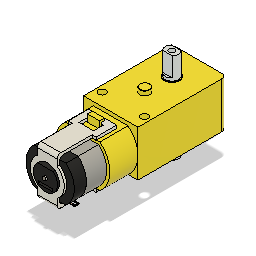
BO DC Motor (Autodesk Fusion 360 design; units mm, degrees)
Autodesk Fusion 360 part; units mm, degrees
sketch "Cylinder profile" plane through (0, 0, 0) normal (0, 1, 0) x (1, 0, 0) in component "Motor Shaft"
  circle A0 centre (0, 0) radius 2.73
  dimension "d6" = 5.46
  measures "d6" diameter of A0
extrude "Extrude1" add sketch "Cylinder profile" along normal mid plane 37.42 makes body 1 in component "Motor Shaft"
sketch "Shaft Cut profile" plane through (0, 18.71, 0) normal (0, 1, 0) x (-1, 0, 0) in component "Motor Shaft"
  circle A0 centre (0, 0) radius 2.73
  line L0 (2.0076, -1.85) -> (-2.0076, -1.85)
  line L1 (0, 0) -> (2.73, 0) construction
  line L2 (2.0076, 1.85) -> (-2.0076, 1.85)
  circle A1 centre (0, 0) radius 1.18
  point P0 (2.73, 0)
  dimension "d9" = 1.85
  dimension "d15" = 2.36
  measures "d9" distance of A0.centre L0
  measures "d15" diameter of A1
extrude "Extrude2" cut sketch "Shaft Cut profile" against normal blind 7.96 contours A0 L2 | A0 L0 bodies 1 in component "Motor Shaft"
extrude "Extrude3" cut sketch "Shaft Cut profile" along normal blind 7.96 from surface at -37.42 contours A0 L2 | A0 L0 bodies 1 in component "Motor Shaft"
extrude "Extrude4" cut sketch "Shaft Cut profile" against normal blind 5.96 contours A1 bodies 1 in component "Motor Shaft"
extrude "Extrude5" cut sketch "Shaft Cut profile" along normal blind 5.96 from surface at -37.42 contours A1 bodies 1 in component "Motor Shaft"
sketch "Case only cross section" plane through (0, 0, 0) normal (0, 1, 0) x (1, 0, 0) in component "Motor Casing"
  circle A0 centre (0, 0) radius 2.73
  line L0 (2.0076, 1.85) -> (-2.0076, 1.85) construction
  line L1 (-2.0076, -1.85) -> (2.0076, -1.85) construction
  line L2 (11.25, 11.33) -> (-11.25, 11.33)
  line L3 (-11.25, 11.33) -> (-11.25, -25.27)
  line L4 (-11.25, -25.27) -> (11.25, -25.27)
  line L5 (11.25, -25.27) -> (11.25, 11.33)
  line L6 (11.25, 11.33) -> (-11.25, -25.27) construction
  line L7 (-11.25, 11.33) -> (11.25, -25.27) construction
  line L8 (0, 9) -> (0, -17) construction
  line L9 (10.25, -21.61) -> (7.25, -21.61) construction
  line L10 (7.25, -21.61) -> (7.25, -18.61) construction
  line L11 (7.25, -18.61) -> (10.25, -18.61) construction
  line L12 (10.25, -18.61) -> (10.25, -21.61) construction
  line L13 (10.25, -21.61) -> (7.25, -18.61) construction
  line L14 (7.25, -21.61) -> (10.25, -18.61) construction
  circle A1 centre (8.75, -20.11) radius 1.5
  circle A2 centre (-8.75, -20.11) radius 1.5
  point P0 (0, -6.97)
  point P1 (8.75, -20.11)
  dimension "d22" = 5.46
  dimension "d37" = 36.6
  dimension "d38" = 22.5
  dimension "d39" = 9.48
  dimension "d41" = 3
  dimension "d42" = 3
  dimension "d44" = 6.66
  dimension "d45" = 4
  dimension "d46" = 3
  measures "d22" diameter of A0
  measures "d37" distance of L2.end L3.end
  measures "d38" distance of L3.end L4.end
  measures "d39" distance of L0 L2
  measures "d41" distance of L10.end L11.end
  measures "d42" distance of L9.end L10.end
  measures "d44" distance of L4 L11
  measures "d45" distance of L5 L10
  measures "d46" diameter of A1
extrude "Extrude1'" add sketch "Case only cross section" along normal mid plane 18.94 separate body makes body 2 in component "Motor Casing"
sketch "Protrusion (wheel side)" plane through (0, 9.47, 0) normal (0, 1, 0) x (-1, 0, 0) in component "Motor Casing"
  circle A0 centre (0, 0) radius 2.73
  circle A1 centre (-8.75, 20.11) radius 1.5
  circle A2 centre (8.75, 20.11) radius 1.5
  line L0 (-11.25, 25.27) -> (-11.25, -11.33)
  line L1 (-11.25, -11.33) -> (11.25, -11.33)
  line L2 (11.25, -11.33) -> (11.25, 25.27)
  line L3 (11.25, 25.27) -> (-11.25, 25.27)
  line L4 (0, -5) -> (0, 13) construction
  line L5 (-2.08, 9.14) -> (2.08, 9.14) construction
  line L6 (2.08, 9.14) -> (2.08, 13.3) construction
  line L7 (2.08, 13.3) -> (-2.08, 13.3) construction
  line L8 (-2.08, 13.3) -> (-2.08, 9.14) construction
  line L9 (-2.08, 9.14) -> (2.08, 13.3) construction
  line L10 (2.08, 9.14) -> (-2.08, 13.3) construction
  line L11 (2.0076, 1.85) -> (-2.0076, 1.85) construction
  circle A3 centre (0, 11.22) radius 2.08
  point P0 (0, 11.22)
  dimension "d50" = 4.16
  dimension "d51" = 4.16
  dimension "d52" = 11.45
  dimension "d53" = 4.16
  measures "d50" distance of L6.end L7.end
  measures "d51" distance of L5.end L6.end
  measures "d52" distance of L7 L11
  measures "d53" diameter of A3
extrude "Extrude2'" add sketch "Protrusion (wheel side)" along normal blind 1.9 contours A3 bodies 2 in component "Motor Casing"
sketch "Casing notch" plane through (0, 0, 0) normal (0, 1, 0) x (1, 0, 0) in component "Motor Casing"
  line L0 (-2.5, 16.53) -> (2.5, 16.53)
  line L1 (2.5, 16.53) -> (2.5, 11.33)
  line L2 (2.5, 11.33) -> (-2.5, 11.33)
  line L3 (-2.5, 11.33) -> (-2.5, 16.53)
  line L4 (11.25, 11.33) -> (-11.25, 11.33) construction
  line L5 (1.5, 12.43) -> (-1.5, 12.43) construction
  line L6 (-1.5, 12.43) -> (-1.5, 15.43) construction
  line L7 (-1.5, 15.43) -> (1.5, 15.43) construction
  line L8 (1.5, 15.43) -> (1.5, 12.43) construction
  line L9 (1.5, 12.43) -> (-1.5, 15.43) construction
  line L10 (-1.5, 12.43) -> (1.5, 15.43) construction
  circle A0 centre (0, 13.93) radius 1.5
  point P0 (0, 13.93)
  dimension "d56" = 5
  dimension "d57" = 5.2
  dimension "d58" = 2.5
  dimension "d60" = 3
  dimension "d61" = 3
  dimension "d62" = 1.1
  dimension "d64" = 3
  measures "d56" distance of L0.start L0.end
  measures "d57" distance of L0.start L2.end
  measures "d58" distance of origin L1
  measures "d60" distance of L6.end L7.end
  measures "d61" distance of L5.end L6.end
  measures "d62" distance of L0 L7
  measures "d64" diameter of A0
extrude "Extrude3'" add sketch "Casing notch" along normal mid plane 3 bodies 2 in component "Motor Casing"
sketch "Motor casing" plane through (0, 0, 25.27) normal (0, 0, 1) x (1, 0, 0) in component "Motor Casing"
  line L0 (11.25, -9.47) -> (11.25, 9.47)
  line L1 (11.25, 9.47) -> (-11.25, 9.47)
  line L2 (-11.25, 9.47) -> (-11.25, -9.47)
  line L3 (-11.25, -9.47) -> (11.25, -9.47)
  line L4 (7.1325, -9.47) -> (-7.1325, -9.47)
  line L5 (0, -0.77) -> (-8, -0.77) construction
  line L6 (7.1325, 7.93) -> (-7.1325, 7.93)
  arc A0 (7.1325, -9.47) -> (7.1325, 7.93) centre (0, -0.77) ccw
  arc A1 (-7.1325, 7.93) -> (-7.1325, -9.47) centre (0, -0.77) ccw
  line L7 (-6.5385, 6.73) -> (6.5385, 6.73)
  line L8 (-6.5385, -8.27) -> (6.5385, -8.27)
  arc A2 (6.5385, -8.27) -> (6.5385, 6.73) centre (0, -0.77) ccw
  arc A3 (-6.5385, 6.73) -> (-6.5385, -8.27) centre (0, -0.77) ccw
  dimension "d74" = 8.7
  dimension "d75" = 11.25
  dimension "d76" = 11.25
  dimension "d82" = 15
  dimension "d83" = 7.5
  dimension "d84" = 9.95
  measures "d74" distance of L5.start L4
  measures "d75" radius of A0
  measures "d76" radius of A1
  measures "d82" distance of L7 L8
  measures "d83" distance of L5.start L8
  measures "d84" radius of A2
extrude "Extrude4'" add sketch "Motor casing" along normal blind 11.6 contours L3 L4 L6 A0 A1 bodies 2 in component "Motor Casing"
sketch "Motor casing rect cutout" plane through (0, 7.93, 0) normal (0, 1, 0) x (-1, 0, 0) in component "Motor Casing"
  line L0 (-7.1325, 25.27) -> (7.1325, 25.27)
  line L1 (7.1325, 25.27) -> (7.1325, 36.87)
  line L2 (7.1325, 36.87) -> (-7.1325, 36.87)
  line L3 (-7.1325, 36.87) -> (-7.1325, 25.27)
  line L4 (-3, 28.87) -> (3, 28.87)
  line L5 (3, 28.87) -> (3, 31.37)
  line L6 (3, 31.37) -> (-3, 31.37)
  line L7 (-3, 31.37) -> (-3, 28.87)
  line L8 (-3, 28.87) -> (3, 31.37) construction
  line L9 (3, 28.87) -> (-3, 31.37) construction
  point P0 (0, 30.12)
  dimension "d90" = 6
  dimension "d91" = 2.5
  dimension "d92" = 3.6
  measures "d90" distance of L5.end L6.end
  measures "d91" distance of L4.end L5.end
  measures "d92" distance of L0 L4
extrude "Extrude5'" cut sketch "Motor casing rect cutout" against normal blind 17.4 contours L4 L5 L6 L7 bodies 2 in component "Motor Casing"
sketch "Motor casing Latch" plane through (0, 0, 0) normal (1, 0, 0) x (0, 0, -1) in component "Motor Casing"
  line L0 (-28.87, 7.93) -> (-31.37, 7.93) construction
  line L1 (-31.37, 7.93) -> (-32.37, 7.93)
  line L2 (-31.37, 7.93) -> (-31.37, 9.93)
  line L3 (-31.37, 9.93) -> (-30.37, 9.93)
  line L4 (-30.37, 9.93) -> (-30.37, 10.93)
  line L5 (-30.37, 10.93) -> (-32.37, 10.93)
  line L6 (-32.37, 10.93) -> (-32.37, 7.93)
  line L7 (-31.37, -9.47) -> (-28.87, -9.47) construction
  line L8 (-31.37, -9.47) -> (-32.37, -9.47)
  line L9 (-31.37, -9.47) -> (-31.37, -11.47)
  line L10 (-31.37, -11.47) -> (-30.37, -11.47)
  line L11 (-30.37, -11.47) -> (-30.37, -12.47)
  line L12 (-30.37, -12.47) -> (-32.37, -12.47)
  line L13 (-32.37, -12.47) -> (-32.37, -9.47)
  dimension "d103" = 1
  dimension "d104" = 2
  dimension "d105" = 1
  dimension "d106" = 1
  dimension "d107" = 2
  dimension "d108" = 1
  dimension "d109" = 2
  dimension "d110" = 1
  dimension "d111" = 1
  dimension "d112" = 2
  measures "d103" distance of L0.end L1.end
  measures "d104" distance of L0.end L2.end
  measures "d105" distance of L2.end L3.end
  measures "d106" distance of L3.end L4.end
  measures "d107" distance of L4.end L5.end
  measures "d108" distance of L7.start L8.end
  measures "d109" distance of L7.start L9.end
  measures "d110" distance of L9.end L10.end
  measures "d111" distance of L10.end L11.end
  measures "d112" distance of L11.end L12.end
extrude "Extrude6" add sketch "Motor casing Latch" along normal mid plane 5 bodies 2 in component "Motor Casing"
fillet "Fillet1" radius 2 2 edges at (-11.25, 0, -11.33) (11.25, 0, -11.33) on bodies 2 in component "Motor Casing"
fillet "Fillet2" radius 1 2 edges at (2.5, 0, -11.33) (-2.5, 0, -11.33) on bodies 2 in component "Motor Casing"
sketch "Motor cross section" plane through (0, 0, 25.27) normal (0, 0, 1) x (1, 0, 0) in component "Driving Motor"
  line L0 (-6.5385, -8.27) -> (6.5385, -8.27)
  arc A0 (6.5385, -8.27) -> (6.5385, 6.73) centre (0, -0.77) ccw
  line L1 (6.5385, 6.73) -> (-6.5385, 6.73)
  arc A1 (-6.5385, 6.73) -> (-6.5385, -8.27) centre (0, -0.77) ccw
extrude "Extrude1''" add sketch "Motor cross section" along normal blind 25 separate body makes body 3 in component "Driving Motor"
ref_plane "WorkPlane1" through (0, -0.77, 45.27) normal (0, 0, 1) x (1, 0, 0) in component "Driving Motor"
split "Split1" by plane through (0, -0.77, 45.27) normal (0, 0, 1) bodies 3 makes body 4 at (1.8819, 0.3568, 50.27) in component "Driving Motor"
sketch "ECT section" plane through (0, -8.27, 0) normal (0, -1, 0) x (1, 0, 0) in component "Driving Motor"
  line L0 (-6.5385, 45.27) -> (6.5385, 45.27) construction
  line L1 (6.5385, 45.27) -> (6.5385, 50.27) construction
  line L2 (6.5385, 50.27) -> (-6.5385, 50.27) construction
  line L3 (-6.5385, 50.27) -> (-6.5385, 45.27) construction
  line L4 (-6.5385, 50.27) -> (6.5385, 45.27) construction
  line L5 (-6.5385, 45.27) -> (6.5385, 50.27) construction
  line L6 (8.6, 48.77) -> (-8.6, 48.77)
  line L7 (-8.6, 48.77) -> (-8.6, 46.77)
  line L8 (-8.6, 46.77) -> (8.6, 46.77)
  line L9 (8.6, 46.77) -> (8.6, 48.77)
  line L10 (8.6, 48.77) -> (-8.6, 46.77) construction
  line L11 (-8.6, 48.77) -> (8.6, 46.77) construction
  line L12 (8.1, 48.27) -> (6.1, 48.27)
  line L13 (6.1, 48.27) -> (6.1, 47.27)
  line L14 (6.1, 47.27) -> (8.1, 47.27)
  line L15 (8.1, 47.27) -> (8.1, 48.27)
  line L16 (8.1, 48.27) -> (6.1, 47.27) construction
  line L17 (6.1, 48.27) -> (8.1, 47.27) construction
  line L18 (0, 45.9618) -> (0, 49.5782) construction
  line L19 (-6.1, 47.27) -> (-8.1, 47.27)
  line L20 (-8.1, 47.27) -> (-8.1, 48.27)
  line L21 (-8.1, 48.27) -> (-6.1, 48.27)
  line L22 (-6.1, 48.27) -> (-6.1, 47.27)
  point P0 (0, 47.77)
  point P1 (7.1, 47.77)
  dimension "d129" = 17.2
  dimension "d130" = 2
  dimension "d132" = 1
  dimension "d133" = 2
  dimension "d134" = 0.5
  measures "d129" distance of L7.end L8.end
  measures "d130" distance of L6.end L7.end
  measures "d132" distance of L12.end L13.end
  measures "d133" distance of L13.end L14.end
  measures "d134" distance of L9 L15
extrude "Extrude2''" add sketch "ECT section" along normal blind 0.25 separate body makes body 5 in component "Driving Motor"
sketch "Motor bottom extension" plane through (0, 0, 50.27) normal (0, 0, 1) x (1, 0, 0) in component "Driving Motor"
  arc A0 (-6.5385, 6.73) -> (-6.5385, -8.27) centre (0, -0.77) ccw construction
  line L0 (-6.5385, -8.27) -> (6.5385, -8.27) construction
  arc A1 (6.5385, -8.27) -> (6.5385, 6.73) centre (0, -0.77) ccw construction
  line L1 (6.5385, 6.73) -> (-6.5385, 6.73) construction
  line L2 (3.2261, 3.05) -> (-3.2261, 3.05)
  arc A2 (-3.2261, 3.05) -> (3.2261, 3.05) centre (0, -0.77) ccw
  line L3 (3, -3.22) -> (-3, -3.22)
  line L4 (-3, -3.22) -> (-3, -4.22)
  line L5 (-3, -4.22) -> (3, -4.22)
  line L6 (3, -4.22) -> (3, -3.22)
  line L7 (3, -3.22) -> (-3, -4.22) construction
  line L8 (-3, -3.22) -> (3, -4.22) construction
  circle A3 centre (0, -0.77) radius 0.75
  point P0 (0, -3.72)
  dimension "d141" = 10
  dimension "d142" = 3.82
  dimension "d143" = 6
  dimension "d144" = 1
  dimension "d145" = 3.45
  dimension "d146" = 1.5
  measures "d141" diameter of A2
  measures "d142" distance of A0.centre L2
  measures "d143" distance of L4.end L5.end
  measures "d144" distance of L3.end L4.end
  measures "d145" distance of A0.centre L5
  measures "d146" diameter of A3
extrude "Extrude3''" add sketch "Motor bottom extension" along normal blind 2 bodies 4 in component "Driving Motor"
extrude "Extrude4''" add 1 faces at (0.3665, -0.77, 50.27) along direction (0, 0, 1) blind 2.5 separate body on bodies 4 makes body 6 in component "Driving Motor"
sketch "Motor Belt (Top)" plane through (0, 7.93, 0) normal (0, 1, 0) x (-1, 0, 0) in component "Fasteners"
  line L0 (-2.5, 31.37) -> (-2.5, 32.37)
  line L1 (-2.5, 32.37) -> (2.5, 32.37) construction
  line L2 (2.5, 32.37) -> (2.5, 31.37)
  line L3 (2.5, 31.37) -> (3, 31.37) construction
  line L4 (3, 31.37) -> (3, 28.87) construction
  line L5 (3, 28.87) -> (-3, 28.87) construction
  line L6 (-3, 28.87) -> (-3, 31.37) construction
  line L7 (-3, 31.37) -> (-2.5, 31.37) construction
  line L8 (-5.75, 28.57) -> (5.75, 28.57)
  line L9 (5.75, 28.57) -> (5.75, 37.07)
  line L10 (-5.75, 37.07) -> (-5.75, 28.57)
  line L11 (-5.75, 28.57) -> (5.75, 37.07) construction
  line L12 (5.75, 28.57) -> (-5.75, 37.07) construction
  line L13 (3, 31.37) -> (-3, 31.37) construction
  line L14 (3, 31.37) -> (-3, 31.37)
  line L15 (-3, 31.37) -> (-3, 35.37)
  line L16 (-3, 35.37) -> (3, 35.37)
  line L17 (3, 35.37) -> (3, 31.37)
  line L18 (-3, 28.87) -> (-3, 31.37) construction
  line L19 (3, 28.87) -> (-3, 28.87) construction
  line L20 (3, 31.37) -> (3, 28.87) construction
  line L21 (4.1, 37.07) -> (4.1, 51.47)
  line L22 (4.1, 51.47) -> (-4.1, 51.47)
  line L23 (-4.1, 51.47) -> (-4.1, 37.07)
  line L24 (-4.1, 37.07) -> (4.1, 51.47) construction
  line L25 (4.1, 37.07) -> (-4.1, 51.47) construction
  line L26 (5.75, 37.07) -> (4.1, 37.07)
  line L27 (-4.1, 37.07) -> (-5.75, 37.07)
  point P0 (0, 32.82)
  point P1 (0, 44.27)
  dimension "d154" = 11.5
  dimension "d155" = 8.5
  dimension "d156" = 0.3
  dimension "d157" = 6
  dimension "d158" = 4
  dimension "d159" = 8.2
  dimension "d160" = 14.4
  measures "d154" distance of L9.end L10.start
  measures "d155" distance of L8.end L9.end
  measures "d156" distance of L5 L8
  measures "d157" distance of L3.end L6.end
  measures "d158" distance of L3.end L16.end
  measures "d159" distance of L21.end L22.end
  measures "d160" distance of L21.start L21.end
sketch "Motor Belt (Bottom)" plane through (0, -9.47, 0) normal (0, -1, 0) x (1, 0, 0) in component "Fasteners"
  line L0 (2.5, 32.37) -> (2.5, 31.37) construction
  line L1 (2.5, 31.37) -> (3, 31.37) construction
  line L2 (3, 31.37) -> (3, 28.87) construction
  line L3 (3, 28.87) -> (-3, 28.87) construction
  line L4 (-3, 28.87) -> (-3, 31.37) construction
  line L5 (-3, 31.37) -> (-2.5, 31.37) construction
  line L6 (-2.5, 31.37) -> (-2.5, 32.37) construction
  line L7 (-2.5, 32.37) -> (2.5, 32.37) construction
  line L8 (5.75, 37.07) -> (5.75, 28.57)
  line L9 (4.1, 51.47) -> (4.1, 37.07)
  line L10 (-4.1, 51.47) -> (4.1, 51.47)
  line L11 (-4.1, 37.07) -> (-4.1, 51.47)
  line L12 (-5.75, 37.07) -> (-4.1, 37.07)
  line L13 (-5.75, 28.57) -> (-5.75, 37.07)
  line L14 (5.75, 28.57) -> (-5.75, 28.57)
  line L15 (4.1, 37.07) -> (5.75, 37.07)
  line L16 (3, 35.37) -> (-3, 35.37)
  line L17 (-3, 35.37) -> (-3, 31.37)
  line L18 (3, 31.37) -> (3, 35.37)
  line L19 (-3, 31.37) -> (3, 31.37)
sketch "ECT Spacer base" plane through (0, -8.52, 0) normal (0, -1, 0) x (1, 0, 0) in component "Fasteners"
  line L0 (4.07, 48.77) -> (-4.07, 48.77)
  line L1 (-4.07, 48.77) -> (-4.07, 45.77)
  line L2 (-4.07, 45.77) -> (4.07, 45.77)
  line L3 (4.07, 45.77) -> (4.07, 48.77)
  line L4 (4.07, 48.77) -> (-4.07, 45.77) construction
  line L5 (-4.07, 48.77) -> (4.07, 45.77) construction
  line L6 (8.6, 48.77) -> (-8.6, 48.77) construction
  point P0 (0, 47.27)
  dimension "d161" = 8.14
  dimension "d162" = 3
  measures "d161" distance of L1.end L2.end
  measures "d162" distance of L0.end L1.end
extrude "Extrude1'''" add sketch "ECT Spacer base" along normal blind 0.7 separate body makes body 7 in component "Fasteners"
extrude "Extrude2'''" add sketch "Motor Belt (Bottom)" along normal blind 1.2 separate body makes body 8 in component "Fasteners"
extrude "Extrude3'''" add sketch "Motor Belt (Top)" along normal blind 1.2 separate body makes body 9 in component "Fasteners"
sketch "Motor belt base" plane through (0, 0, 51.47) normal (0, 0, 1) x (1, 0, 0) in component "Fasteners"
  line L0 (4.1, -9.47) -> (-4.1, -9.47)
  line L1 (-4.1, -9.47) -> (-4.1, -10.67)
  line L2 (-4.1, -10.67) -> (4.1, -10.67)
  line L3 (4.1, -10.67) -> (4.1, -9.47)
  line L4 (-4.1, 7.93) -> (4.1, 7.93)
  line L5 (4.1, -9.47) -> (-4.1, -9.47)
  arc A0 (-3.2261, 3.05) -> (3.2261, 3.05) centre (0, -0.77) ccw construction
  circle A1 centre (0, -0.77) radius 5
  line L6 (-4.1, 4.9036) -> (-4.1, 7.93)
  line L7 (4.1, 7.93) -> (4.1, 4.9036)
  line L8 (4.1, 2.0918) -> (4.1, -3.6318)
  line L9 (4.1, -6.4436) -> (4.1, -9.47)
  line L10 (-4.1, -9.47) -> (-4.1, -6.4436)
  line L11 (-4.1, -3.6318) -> (-4.1, 2.0918)
  arc A2 (-4.1, 4.9036) -> (-4.1, -6.4436) centre (0, -0.77) ccw
  arc A3 (4.1, -6.4436) -> (4.1, 4.9036) centre (0, -0.77) ccw
  point P0 (-4.1, 7.93)
  dimension "d169" = 14
  measures "d169" diameter of A2
extrude "Extrude4'''" add sketch "Motor belt base" against normal blind 1 contours L0 L4 L5 L6 L7 L9 L10 A2 A3 bodies 8 9 in component "Fasteners"
fillet "Fillet1'" radius 1.5 4 edges at (0, 9.13, 51.47) (0, -10.67, 51.47) (0, -9.47, 50.47) (0, 7.93, 50.47) on bodies 8 in component "Fasteners"
sketch "Sketch12" plane through (0, 9.47, 0) normal (0, 1, 0) x (-1, 0, 0) in component "Motor Casing"
  arc A0 (-11.25, -9.33) -> (-9.25, -11.33) centre (-9.25, -9.33) ccw
  line L0 (-9.25, -11.33) -> (9.25, -11.33)
  arc A1 (9.25, -11.33) -> (11.25, -9.33) centre (9.25, -9.33) ccw
  line L1 (11.25, -9.33) -> (11.25, 25.27)
  line L2 (11.25, 25.27) -> (-11.25, 25.27)
  line L3 (-11.25, 25.27) -> (-11.25, -9.33)
  circle A2 centre (0, 11.22) radius 2.08
  circle A3 centre (0, 0) radius 2.73
  circle A4 centre (-8.75, 20.11) radius 1.5
  circle A5 centre (8.75, 20.11) radius 1.5
  circle A6 centre (0, 0) radius 2.73
  circle A7 centre (0, 0) radius 3.2
  dimension "d173" = 6.4
  measures "d173" diameter of A7
extrude "Extrude7" add sketch "Sketch12" along normal blind 0.15 contours A7 bodies 2 in component "Motor Casing"
chamfer "Chamfer1" distance 0.15 angle 45 1 edges at (1.9392, 11.37, 10.4678) on bodies 2 in component "Motor Casing"
fillet "Fillet3" radius 0.15 1 edges at (2.9834, 9.62, -1.1572) on bodies 2 in component "Motor Casing"
component "Motor Shaft" placed x (1, 0, 0) y (0, 1, 0) z (0, 0, 1) at (0, 0, 0)
component "Motor Casing" placed x (1, 0, 0) y (0, 1, 0) z (0, 0, 1) at (0, 0, 0)
component "Driving Motor" placed x (1, 0, 0) y (0, 1, 0) z (0, 0, 1) at (0, 0, 0)
component "Fasteners" placed x (1, 0, 0) y (0, 1, 0) z (0, 0, 1) at (0, 0, 0)
equation "SHAFT_DIAMETER_EXTERNAL = 5.46 mm" comment "The external diameter of shaft"
equation "SHAFT_WIDTH_CUT = 3.70 mm" comment "Width of the top section of shaft with cut"
equation "SHAFT_LENGTH = 37.42 mm" comment "Length of shaft"
equation "SHAFT_CUT_LENGTH = 7.96 mm" comment "Length from top surface for the cut section"
equation "SHAFT_DIAMETER_INNER = 2.36 mm" comment "Inner circle diameter of shaft"
equation "d6 = SHAFT_DIAMETER_EXTERNAL"
equation "d7 = SHAFT_LENGTH / 2"
equation "d9 = SHAFT_WIDTH_CUT / 2"
equation "d10 = -SHAFT_CUT_LENGTH"
equation "d13 = SHAFT_CUT_LENGTH"
equation "d15 = SHAFT_DIAMETER_INNER"
equation "SHAFT_INNER_HOLE_DEPTH = SHAFT_CUT_LENGTH - 2 mm" comment "The depth of the internal holes in the shaft"
equation "d17 = -SHAFT_INNER_HOLE_DEPTH"
equation "d20 = SHAFT_INNER_HOLE_DEPTH"
equation "d22 = SHAFT_DIAMETER_EXTERNAL"
equation "CASING_WOM_LENGTH = 36.6 mm" comment "Length of casing without motor mount"
equation "CASING_WIDTH = 22.5 mm" comment "Width of the casing"
equation "CASING_WOM_DEPTH = 18.94 mm" comment "Depth of the case without motor mount"
equation "CASING_PROTRUSION_HEIGHT_FROM_BASE = 20.84 mm" comment "Height from base to protrusion top for the casing"
equation "CASING_PRO_HEIGHT = CASING_PROTRUSION_HEIGHT_FROM_BASE - CASING_WOM_DEPTH" comment "Just the protrusion height for the casing"
equation "CASING_PRO_DIAMETER = 4.16 mm" comment "Diameter of the protrusion from the case (which is towards the wheel)"
equation "CASING_PRO_SHAFT_B_TO_B = 11.45 mm" comment "The length from bottom of the protrusion to the horizontal bottom cut of the shaft."
equation "CASING_WOM_SCREW_HOLE_DIA = 3 mm" comment "The screw hole diameter of the casing (without motor)"
equation "CASING_WOM_SCREW_HOLE_BOTTOM_TOP = 6.66 mm" comment "Distance from top of the screw support hole to the bottom of the case without motor casing"
equation "CASING_WOM_SCREW_HOLE_EDGE = 4 mm" comment "Maximum distance from the screw hole edge to the casing vertical edge"
equation "CASING_NOTCH_DEPTH = 3 mm" comment "The depth of the top notch in the casing"
equation "CASING_NOTCH_WIDTH = 5 mm" comment "The width of notch above casing"
equation "CASING_NOTCH_HEIGHT = 5.2 mm" comment "THe height of notch on the top of casing"
equation "CASING_WOM_SHAFT_TOP_TO_TOP = 9.48 mm" comment "The distance from the top of the flat motor shaft to casing top (from where the notch starts)"
equation "d37 = CASING_WOM_LENGTH"
equation "d38 = CASING_WIDTH"
equation "d39 = CASING_WOM_SHAFT_TOP_TO_TOP"
equation "d41 = CASING_WOM_SCREW_HOLE_DIA"
equation "d42 = CASING_WOM_SCREW_HOLE_DIA"
equation "d44 = CASING_WOM_SCREW_HOLE_BOTTOM_TOP"
equation "d45 = CASING_WOM_SCREW_HOLE_EDGE"
equation "d46 = CASING_WOM_SCREW_HOLE_DIA"
equation "d47 = CASING_WOM_DEPTH"
equation "d50 = CASING_PRO_DIAMETER"
equation "d51 = CASING_PRO_DIAMETER"
equation "d52 = CASING_PRO_SHAFT_B_TO_B"
equation "d53 = CASING_PRO_DIAMETER"
equation "d54 = CASING_PRO_HEIGHT"
equation "d56 = CASING_NOTCH_WIDTH"
equation "d57 = CASING_NOTCH_HEIGHT"
equation "d58 = CASING_NOTCH_WIDTH / 2.0"
equation "CASING_NOTCH_HOLE_DIA = 3 mm" comment "The diameter of the hole in the notch"
equation "d60 = CASING_NOTCH_HOLE_DIA"
equation "d61 = CASING_NOTCH_HOLE_DIA"
equation "d62 = CASING_NOTCH_HOLE_MD"
equation "CASING_NOTCH_HOLE_MD = 1.1 mm" comment "The distance from the top of hole in notch to absolute top of notch"
equation "d64 = CASING_NOTCH_HOLE_DIA"
equation "d65 = CASING_NOTCH_DEPTH"
equation "MCASE_W_EXT = 22.5 mm" comment "The external width of the motor casing"
equation "MCASE_W_INT = 19.9 mm" comment "The internal width of the motor casing"
equation "MCASE_H_EXT = 17.4 mm" comment "The external height of the motor casing"
equation "MCASE_H_INT = 15 mm" comment "The internal height of the motor casing"
equation "MCASE_L = 11.6 mm" comment "The length of motor casing"
equation "d74 = MCASE_H_EXT / 2"
equation "d75 = MCASE_W_EXT / 2"
equation "d76 = d75"
equation "d82 = MCASE_H_INT"
equation "d83 = MCASE_H_INT / 2"
equation "d84 = MCASE_W_INT / 2"
equation "d85 = MCASE_L"
equation "MCASE_RHOLE_H = 2.5 mm" comment "The height of the cutout in the motor case (under motor belt)"
equation "MCASE_RHOLE_W = 6 mm" comment "The width of the rectangular cutout in the motor casing (under the motor belt)"
equation "MCASE_RHOLE_TOP = 3.6 mm" comment "The distance from the top of the motor housing to the top of the rectangular cutout"
equation "d90 = MCASE_RHOLE_W"
equation "d91 = MCASE_RHOLE_H"
equation "d92 = MCASE_RHOLE_TOP"
equation "MCASE_LS_T = 1 mm" comment "The thickness of the L section for the belt in the motor case"
equation "MCASE_LS_H = 2 mm" comment "The height of L section of motor case (for belt)"
equation "MCASE_LS_W = 1 mm" comment "The width of the L section for the belt (on motor casing)"
equation "d103 = MCASE_LS_T"
equation "d104 = MCASE_LS_H"
equation "d105 = MCASE_LS_W"
equation "d106 = MCASE_LS_W"
equation "d107 = MCASE_LS_W + MCASE_LS_T"
equation "d108 = MCASE_LS_T"
equation "d109 = MCASE_LS_H"
equation "d110 = MCASE_LS_W"
equation "d111 = MCASE_LS_T"
equation "d112 = MCASE_LS_W + MCASE_LS_T"
equation "MCASE_LS_TW = 5 mm" comment "The width of the L section on motor casing (as seen from top view)"
equation "d114 = MCASE_LS_TW"
equation "d116 = CASING_TOPC_FR"
equation "CASING_TOPC_FR = 2 mm" comment "Fillet radius of the top edge (top face) along the axis of shaft"
equation "d118 = CASING_TOPN_FR"
equation "CASING_TOPN_FR = 1 mm" comment "Fillet radius for the base of the notch"
equation "MOTOR_L = 25 mm" comment "Length of motor"
equation "d121 = MOTOR_L"
equation "MOTOR_CONT_L = 5 mm" comment "Length of motor connection terminals"
equation "d124 = -MOTOR_CONT_L"
equation "MOTOR_ECT_W = 2 mm" comment "Width of electrical connection terminal (ECT) on motor"
equation "MOTOR_ECT_L = 17.2 mm" comment "Length of the electrical connection terminal on the motor"
equation "MOTOR_ECT_RH_W = MOTOR_ECT_W" comment "The width of the rectangular hole in the ECT"
equation "MOTOR_ECT_RH_SEPDIST = 0.5 mm" comment "The separation distance of the rectangular holes on the ECT"
equation "d129 = MOTOR_ECT_L"
equation "d130 = MOTOR_ECT_W"
equation "MOTOR_ECT_RH_H = 1 mm" comment "The height of the hole in the ECT of motor"
equation "d132 = MOTOR_ECT_RH_H"
equation "d133 = MOTOR_ECT_RH_W"
equation "d134 = MOTOR_ECT_RH_SEPDIST"
equation "MOTOR_ECT_D = 0.25 mm" comment "The thickness of the ECT connected to motor"
equation "d136 = MOTOR_ECT_D"
equation "MOTOR_BOTTOM_D = 10 mm" comment "The diameter of the bottom extension of motor"
equation "MOTOR_BOTTOM_L = 2 mm" comment "The length of the bottom section of motor"
equation "MOTOR_BOTTOM_CSD = 8.82 mm" comment "The distance (Cut Section Distance)of the top flat of the bottom of motor to the bottom of the circular bottom base"
equation "d141 = MOTOR_BOTTOM_D"
equation "d142 = MOTOR_BOTTOM_CSD - MOTOR_BOTTOM_D / 2"
equation "d147 = MOTOR_BOTTOM_L"
equation "d149 = MOTOR_BOTTOM_PIN_L"
equation "MOTOR_BOTTOM_PIN_L = 2.5 mm" comment "The length of motor shaft pin at the bottom"
named bodies: "Main Motor Shaft", "Casing w/o motor case", "Aluminium section", "Connection section", "Motor ECT", "Motor bottom shaft pin", "Motor ECT spacer", "Motor belt"
